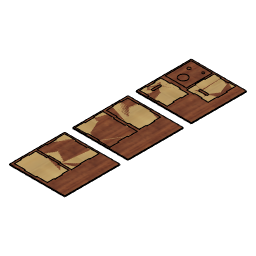
PLYO BOX v15 (Autodesk Fusion 360 design; units mm, degrees)
Autodesk Fusion 360 part; units mm, degrees
sketch "Sketch1" plane through (0, 0, 0) normal (0, 1, 0) x (1, 0, 0)
  line L0 (381, 304.8) -> (-381, 304.8)
  line L1 (-381, 304.8) -> (-381, -304.8)
  line L2 (-381, -304.8) -> (381, -304.8)
  line L3 (381, -304.8) -> (381, 304.8)
  line L4 (381, 304.8) -> (-381, -304.8) construction
  line L5 (-381, 304.8) -> (381, -304.8) construction
  line L6 (-127, 304.8) -> (127, 304.8)
  line L7 (127, 304.8) -> (127, 286.8)
  line L8 (127, 286.8) -> (-127, 286.8)
  line L9 (-127, 286.8) -> (-127, 304.8)
  line L10 (0, -304.8) -> (0, 304.8) construction
  line L11 (381, 0) -> (-381, 0) construction
  line L12 (127, -286.8) -> (-127, -286.8)
  line L13 (127, -304.8) -> (127, -286.8)
  line L14 (-127, -286.8) -> (-127, -304.8)
  line L15 (-381, -101.6) -> (-363, -101.6)
  line L16 (-363, -101.6) -> (-363, 101.6)
  line L17 (-363, 101.6) -> (-381, 101.6)
  line L18 (-381, 101.6) -> (-381, -101.6)
  line L19 (363, -101.6) -> (363, 101.6)
  line L20 (381, -101.6) -> (363, -101.6)
  line L21 (363, 101.6) -> (381, 101.6)
  dimension "Breedte" = 762
  dimension "Hoogte" = 609.6
  dimension "d3" = 254
  dimension "diktehout" = 18
  dimension "d5" = 203.2
  dimension "d6" = 18
  constraint horizontal L0
  constraint perpendicular L0 L1
  constraint parallel L0 L2
  constraint parallel L1 L3
  constraint coincident L4 origin
  constraint coincident L5 origin
  constraint horizontal L6
  constraint vertical L7
  constraint horizontal L8
  constraint vertical L9
  constraint coincident L0 L6.start
  constraint midpoint L2 L10.start
  constraint midpoint L0 L10.end
  constraint midpoint L3 L11.start
  constraint midpoint L1 L11.end
  constraint symmetric L7 L9 L10
  constraint symmetric L6.start L11 L14.end
  constraint symmetric L6.end L11 L13.start
  constraint symmetric L7.end L11 L12.start
  constraint symmetric L8.end L11 L12.end
  constraint horizontal L15
  constraint vertical L16
  constraint horizontal L17
  constraint vertical L18
  constraint coincident L1 L15.start
  constraint symmetric L11 L15 L17
  constraint symmetric L10 L15.start L20.start
  constraint symmetric L10 L15.end L19.start
  constraint symmetric L10 L16.end L19.end
  constraint symmetric L10 L17.end L21.end
  measures "Breedte" distance of L0.start L0.end
  measures "Hoogte" distance of L0.start L2.end
  measures "d3" distance of L7.end L8.end
  measures "diktehout" distance of L6.end L7.end
  measures "d5" distance of L15.end L16.end
  measures "d6" distance of L16.end L17.end
extrude "Extrude1" add sketch "Sketch1" along normal blind 18 contours L0 L1 L2 L3 L7 L8 L9 L12 L13 L14 L15 L16 L17 L19 L20 L21 makes body 1 in component "Voorkant"
sketch "Sketch1 (2)" plane through (381, 0, 0) normal (1, 0, 0) x (0, 1, 0) in component "zijkant"
  line L0 (0, 304.8) -> (0, 101.6)
  line L1 (0, 101.6) -> (18, 101.6)
  line L2 (18, 101.6) -> (18, 304.8)
  line L3 (18, 304.8) -> (0, 304.8)
  line L4 (18, 304.8) -> (-490, 304.8)
  line L5 (-490, 304.8) -> (-490, -304.8)
  line L6 (-490, -304.8) -> (18, -304.8)
  line L7 (18, -304.8) -> (18, 304.8)
  line L8 (18, 304.8) -> (0, 304.8)
  line L9 (0, 304.8) -> (0, -304.8)
  line L10 (0, -304.8) -> (18, -304.8)
  line L11 (18, -304.8) -> (18, 304.8)
  line L12 (18, -101.6) -> (0, -101.6)
  line L13 (18, 101.6) -> (0, 101.6)
  line L14 (-236, 304.8) -> (-236, -304.8) construction
  line L15 (-472, 304.8) -> (-472, -304.8)
  line L16 (-490, 101.6) -> (-472, 101.6)
  line L17 (-490, -101.6) -> (-472, -101.6)
  line L18 (-320.6667, 304.8) -> (-151.3333, 304.8)
  line L19 (-151.3333, 304.8) -> (-151.3333, 286.8)
  line L20 (-151.3333, 286.8) -> (-320.6667, 286.8)
  line L21 (-320.6667, 286.8) -> (-320.6667, 304.8)
  line L22 (18, 0) -> (-490, 0) construction
  line L23 (-151.3333, -286.8) -> (-320.6667, -286.8)
  line L24 (-320.6667, -286.8) -> (-320.6667, -304.8)
  line L25 (-151.3333, -304.8) -> (-151.3333, -286.8)
  dimension "d9" = 609.6
  dimension "Diepte" = 508
  dimension "d11" = 18
  dimension "d12" = 203.2
  dimension "d13" = 203.2
  dimension "d14" = 169.3333
  dimension "d15" = 18
  dimension "d92" = 0
  dimension "d93" = 0
  dimension "d94" = 0
  dimension "d95" = 0
  dimension "d104" = 0
  dimension "d105" = 0
  dimension "d106" = 0
  dimension "d107" = 0
  dimension "d156" = 0
  dimension "d157" = 0
  dimension "d158" = 0
  dimension "d159" = 0
  dimension "d172" = 0
  dimension "d173" = 0
  dimension "d174" = 0
  dimension "d175" = 0
  dimension "d180" = 0
  dimension "d181" = 0
  dimension "d182" = 0
  dimension "d183" = 0
  constraint horizontal L4
  constraint vertical L5
  constraint horizontal L6
  constraint vertical L7
  constraint coincident L2.end L3.start
  constraint horizontal L8
  constraint vertical L9
  constraint horizontal L10
  constraint vertical L11
  constraint coincident L6 L9.end
  constraint coincident L7 L12.start
  constraint coincident L9 L12.end
  constraint perpendicular L7 L12
  constraint coincident L1.end L2.start
  constraint coincident L0.end L1.start
  constraint midpoint L4 L14.start
  constraint midpoint L6 L14.end
  constraint symmetric L0.start L14 L15.start
  constraint symmetric L9.end L14 L15.end
  constraint symmetric L12.start L14 L17.start
  constraint symmetric L12.end L14 L17.end
  constraint symmetric L1.end L14 L16.start
  constraint symmetric L0.end L14 L16.end
  constraint horizontal L18
  constraint vertical L19
  constraint horizontal L20
  constraint vertical L21
  constraint coincident L4 L18.start
  constraint symmetric L14 L19 L21
  constraint midpoint L7 L22.start
  constraint midpoint L5 L22.end
  constraint symmetric L18.start L22 L24.end
  constraint symmetric L18.end L22 L25.start
  constraint symmetric L19.end L22 L23.start
  constraint symmetric L20.end L22 L23.end
  measures "d9" distance of L4.end L5.end
  measures "Diepte" distance of L2.end L4.end
  measures "d11" distance of L9.end L6.end
  measures "d12" distance of L4 L13
  measures "d13" distance of L10 L12
  measures "d14" distance of L19.end L20.end
  measures "d15" distance of L18.end L19.end
extrude "Extrude1'" add sketch "Sketch1 (2)" along normal blind 18 separate body contours L0 L4 L6 L9 L15 L19 L20 L21 L23 L24 L25 makes body 2 in component "Middenstuk"
extrude "Extrude1''" add sketch "Sketch1 (2)" against normal blind 18 separate body contours L0 L4 L6 L9 L15 L19 L20 L21 L23 L24 L25 | L1 L7 L9 L11 L12 L13 | L5 L15 L16 L17 makes body 3 in component "zijkant"
sketch "Sketch1 (3)" plane through (0, 0, -304.8) normal (0, 0, -1) x (1, 0, 0) in component "Onderkant"
  line L0 (-127, 0) -> (-381, 0)
  line L1 (-381, 0) -> (-381, -18)
  line L2 (-381, -18) -> (-127, -18)
  line L3 (-127, -18) -> (-127, 0)
  line L4 (381, -18) -> (-381, -18)
  line L5 (-381, -18) -> (-381, 490)
  line L6 (-381, 490) -> (381, 490)
  line L7 (381, 490) -> (381, -18)
  line L8 (363, 0) -> (-363, 0)
  line L9 (-363, 0) -> (-363, 472)
  line L10 (-363, 472) -> (363, 472)
  line L11 (363, 472) -> (363, 0)
  line L12 (127, 472) -> (127, 490)
  line L13 (-363, 151.3333) -> (-381, 151.3333)
  line L14 (-363, 320.6667) -> (-381, 320.6667)
  line L15 (-127, 472) -> (-127, 490)
  line L16 (0, -18) -> (0, 490) construction
  line L17 (-381, 236) -> (381, 236) construction
  line L18 (-127, 0) -> (-127, -18)
  line L19 (127, 0) -> (127, -18)
  line L20 (363, 151.3333) -> (381, 151.3333)
  line L21 (363, 320.6667) -> (381, 320.6667)
  point P0 (381, -18)
  dimension "d18" = 508
  dimension "d19" = 762
  dimension "d20" = 18
  dimension "d22" = 254
  dimension "d23" = 169.3333
  dimension "d60" = 0
  dimension "d61" = 0
  dimension "d62" = 0
  dimension "d63" = 0
  dimension "d72" = 0
  dimension "d73" = 0
  dimension "d74" = 0
  dimension "d75" = 0
  dimension "d80" = 0
  dimension "d81" = 0
  dimension "d82" = 0
  dimension "d83" = 0
  dimension "d132" = 0
  dimension "d133" = 0
  dimension "d134" = 0
  dimension "d135" = 0
  dimension "d140" = 0
  dimension "d141" = 0
  dimension "d142" = 0
  dimension "d143" = 0
  dimension "d148" = 0
  dimension "d149" = 0
  dimension "d150" = 0
  dimension "d151" = 0
  dimension "d164" = 0
  dimension "d165" = 0
  dimension "d166" = 0
  dimension "d167" = 0
  dimension "d188" = 0
  dimension "d189" = 0
  dimension "d190" = 0
  dimension "d191" = 0
  dimension "d196" = 0
  dimension "d197" = 0
  dimension "d198" = 0
  dimension "d199" = 0
  dimension "d220" = 0
  dimension "d221" = 0
  dimension "d222" = 0
  dimension "d223" = 0
  constraint horizontal L4
  constraint vertical L5
  constraint horizontal L6
  constraint vertical L7
  constraint coincident P0 L4.start
  constraint coincident L10 L12.start
  constraint coincident L6 L12.end
  constraint perpendicular L6 L12
  constraint coincident L9 L13.start
  constraint coincident L5 L13.end
  constraint perpendicular L5 L13
  constraint coincident L9 L14.start
  constraint coincident L5 L14.end
  constraint perpendicular L5 L14
  constraint coincident L10 L15.start
  constraint coincident L6 L15.end
  constraint perpendicular L6 L15
  constraint midpoint L4 L16.start
  constraint midpoint L6 L16.end
  constraint midpoint L5 L17.start
  constraint midpoint L7 L17.end
  constraint symmetric L13 L14 L17
  constraint symmetric L12 L15 L16
  constraint symmetric L12.start L17 L19.start
  constraint symmetric L12.end L17 L19.end
  constraint symmetric L15.start L17 L0.start
  constraint symmetric L15.end L17 L2.end
  constraint symmetric L13.start L16 L20.start
  constraint symmetric L13.end L16 L20.end
  constraint symmetric L14.start L16 L21.start
  constraint symmetric L14.end L16 L21.end
  measures "d18" distance of L1.end L5.end
  measures "d19" distance of L5.end L6.end
  measures "d22" distance of L12 L15
  measures "d23" distance of L13 L14
extrude "Extrude1'''" add sketch "Sketch1 (3)" against normal blind 18 separate body contours L3 L4 L8 L18 L19 | L0 L8 L9 L10 L11 | L5 L9 L13 L14 | L7 L11 L20 L21 | L6 L10 L12 L15 makes body 4 in component "Onderkant"
extrude "Extrude2" cut 2 faces at (387, -421.5556, -304.8) (387, -100.8889, -304.8) along direction (0, 0, -1) up to surface end surface through (381, -151.3333, -286.8) normal (0, 0, -1) offset 0 on bodies 2 bodies 2 in component "Middenstuk"
extrude "Extrude3" cut 2 faces at (387, -371.1111, 304.8) (387, -50.4444, 304.8) along direction (0, 0, 1) up to surface end surface through (381, -151.3333, 286.8) normal (0, 0, 1) offset 0 on bodies 2 bodies 2 in component "Middenstuk"
sketch "Sketch1 (4)" plane through (0, 0, 0) normal (0, 0, 1) x (1, 0, 0) in component "Houtplaat"
  line L0 (0, 0) -> (1220, 0)
  line L1 (1220, 0) -> (1220, -1220)
  line L2 (1220, -1220) -> (0, -1220)
  line L3 (0, -1220) -> (0, 0)
  dimension "d32" = 1220
  dimension "d33" = 1220
  dimension "d40" = 0
  dimension "d41" = 0
  dimension "d42" = 0
  dimension "d43" = 0
  dimension "d52" = 0
  dimension "d53" = 0
  dimension "d54" = 0
  dimension "d55" = 0
  dimension "d64" = 0
  dimension "d65" = 0
  dimension "d66" = 0
  dimension "d67" = 0
  dimension "d76" = 0
  dimension "d77" = 0
  dimension "d78" = 0
  dimension "d79" = 0
  dimension "d84" = 0
  dimension "d85" = 0
  dimension "d86" = 0
  dimension "d87" = 0
  dimension "d96" = 0
  dimension "d97" = 0
  dimension "d98" = 0
  dimension "d99" = 0
  dimension "d108" = 0
  dimension "d109" = 0
  dimension "d110" = 0
  dimension "d111" = 0
  dimension "d120" = 0
  dimension "d121" = 0
  dimension "d122" = 0
  dimension "d123" = 0
  dimension "d128" = 0
  dimension "d129" = 0
  dimension "d130" = 0
  dimension "d131" = 0
  dimension "d136" = 0
  dimension "d137" = 0
  dimension "d138" = 0
  dimension "d139" = 0
  dimension "d144" = 0
  dimension "d145" = 0
  dimension "d146" = 0
  dimension "d147" = 0
  dimension "d152" = 0
  dimension "d153" = 0
  dimension "d154" = 0
  dimension "d155" = 0
  dimension "d160" = 0
  dimension "d161" = 0
  dimension "d162" = 0
  dimension "d163" = 0
  dimension "d168" = 0
  dimension "d169" = 0
  dimension "d170" = 0
  dimension "d171" = 0
  dimension "d176" = 0
  dimension "d177" = 0
  dimension "d178" = 0
  dimension "d179" = 0
  dimension "d184" = 0
  dimension "d185" = 0
  dimension "d186" = 0
  dimension "d187" = 0
  dimension "d192" = 0
  dimension "d193" = 0
  dimension "d194" = 0
  dimension "d195" = 0
  dimension "d200" = 0
  dimension "d201" = 0
  dimension "d202" = 0
  dimension "d203" = 0
  dimension "d224" = 0
  dimension "d225" = 0
  dimension "d226" = 0
  dimension "d227" = 0
  constraint horizontal L0
  constraint vertical L1
  constraint horizontal L2
  constraint vertical L3
  constraint coincident L0.start L3.end
  measures "d32" distance of L0.start L2.end
  measures "d33" distance of L1.end L2.end
extrude "Extrude1''''" add sketch "Sketch1 (4)" along normal blind 18 separate body makes body 5 in component "Houtplaat"
sketch "Sketch2" plane through (381, 0, 0) normal (1, 0, 0) x (0, 1, 0)
  line L0 (18, -101.6) -> (18, 101.6)
  line L1 (18, 101.6) -> (0, 101.6)
  line L2 (0, 101.6) -> (0, 304.8)
  line L3 (0, 304.8) -> (-151.3333, 304.8)
  line L4 (-151.3333, 304.8) -> (-151.3333, 286.8)
  line L5 (-151.3333, 286.8) -> (-320.6667, 286.8)
  line L6 (-320.6667, 286.8) -> (-320.6667, 304.8)
  line L7 (-320.6667, 304.8) -> (-472, 304.8)
  line L8 (-472, 304.8) -> (-472, 101.6)
  line L9 (-472, 101.6) -> (-490, 101.6)
  line L10 (-490, 101.6) -> (-490, -101.6)
  line L11 (-490, -101.6) -> (-472, -101.6)
  line L12 (-472, -101.6) -> (-472, -304.8)
  line L13 (-472, -304.8) -> (-320.6667, -304.8)
  line L14 (-320.6667, -304.8) -> (-320.6667, -286.8)
  line L15 (-320.6667, -286.8) -> (-151.3333, -286.8)
  line L16 (-151.3333, -286.8) -> (-151.3333, -304.8)
  line L17 (-151.3333, -304.8) -> (0, -304.8)
  line L18 (0, -304.8) -> (0, -101.6)
  line L19 (0, -101.6) -> (18, -101.6)
  line L20 (-311, 141.8) -> (-161, 141.8)
  arc A0 (-161, 141.8) -> (-161, 191.8) centre (-161, 166.8) ccw
  line L21 (-161, 191.8) -> (-311, 191.8)
  arc A1 (-311, 191.8) -> (-311, 141.8) centre (-311, 166.8) ccw
  line L22 (-311, 166.8) -> (-161, 166.8) construction
  point P0 (-236, 166.8)
  dimension "d268" = 50
  dimension "d269" = 120
  constraint tangent L20 A0
  constraint tangent A0 L21
  constraint parallel L20 L21
  constraint tangent L21 A1
  constraint tangent L20 A1
  constraint parallel L5 L22
  constraint midpoint L22 P0
  measures "d268" diameter of A0
  measures "d269" distance of L5 P0
extrude "Extrude2'" cut sketch "Sketch2" against normal blind 50 contours L20 A0 L21 A1 bodies 3 in component "zijkant"
sketch "Sketch3" plane through (27, 0, 0) normal (1, 0, 0) x (0, 1, 0)
  line L0 (0, 286.8) -> (-472, 286.8)
  line L1 (-472, 286.8) -> (-472, -286.8)
  line L2 (-472, -286.8) -> (0, -286.8)
  line L3 (0, -286.8) -> (0, 286.8)
  circle A0 centre (-236, -121.8) radius 92.5
  circle A1 centre (-347, 116.8) radius 35
  circle A2 centre (-105, 186.8) radius 25
  line L4 (-236, -286.8) -> (-236, 286.8) construction
  dimension "d272" = 185
  dimension "d273" = 70
  dimension "d274" = 50
  dimension "d275" = 165
  dimension "d276" = 125
  dimension "d277" = 170
  dimension "d278" = 105
  dimension "d279" = 100
  constraint midpoint L2 L4.start
  constraint midpoint L0 L4.end
  constraint coincident A0.centre L4
  measures "d272" diameter of A0
  measures "d273" diameter of A1
  measures "d274" diameter of A2
  measures "d275" distance of L2 A0.centre
  measures "d276" distance of L1 A1.centre
  measures "d277" distance of L0 A1.centre
  measures "d278" distance of L3 A2.centre
  measures "d279" distance of L0 A2.centre
extrude "Extrude4" cut sketch "Sketch3" against normal up to surface (18 mm away) contours A0 | A1 | A2 sketch seen with x (1, 0, 0) y (0, 1, 0) z (0, 0, 1) at (372, 0, 0) bodies 2 in component "Middenstuk"
ref_plane "WorkPlane1" through (27, -236, 0) normal (1, 0, 0) x (0, 0, -1) in component "Laser Path - Middenstuk - Body1"
sketch "Path Offsets" plane through (27, 0, 0) normal (1, 0, 0) x (0, 0, -1) in component "Laser Path - Middenstuk - Body1"
  circle A0 centre (121.8, -236) radius 92.5
  circle A1 centre (-116.8, -347) radius 35
  circle A2 centre (-186.8, -105) radius 25
  line L0 (-286.8, 0) -> (-286.8, -472)
  line L1 (-286.8, -472) -> (286.8, -472)
  line L2 (286.8, -472) -> (286.8, 0)
  line L3 (286.8, 0) -> (-286.8, 0)
  line L4 (-286.8, -472) -> (286.8, -472)
  line L5 (286.8, -472) -> (286.8, 0)
  line L6 (286.8, 0) -> (-286.8, 0)
  line L7 (-286.8, 0) -> (-286.8, -472)
  dimension "d292" = 0
  measures "d292" distance of L1
sketch "Perimeter" plane through (27, -236, 0) normal (1, 0, 0) x (0, 0, -1) in component "Laser Path - Middenstuk - Body1"
  line L0 (286.8, 236) -> (-286.8, 236)
  line L1 (-286.8, 236) -> (-286.8, -236)
  line L2 (-286.8, -236) -> (286.8, -236)
  line L3 (286.8, -236) -> (286.8, 236)
sketch "Cutouts" plane through (27, -236, 0) normal (1, 0, 0) x (0, 0, -1) in component "Laser Path - Middenstuk - Body1"
  circle A0 centre (121.8, 0) radius 92.5
  circle A1 centre (-116.8, -111) radius 35
  circle A2 centre (-186.8, 131) radius 25
component "Voorkant" placed x (1, 0, 0) y (0, 0, 1) z (0, -1, 0) at (409, -1735.2, 0)
component "zijkant" placed x (0, 0, 1) y (0, 1, 0) z (-1, 0, 0) at (330, 702, -363)
component "Onderkant" placed x (1, 0, 0) y (0, 1, 0) z (0, 0, 1) at (409, -2083, 304.8)
component "Onderkant" placed x (1, 0, 0) y (0, 1, 0) z (0, 0, 1) at (406, -48, 304.8)
component "zijkant" placed x (0, 0, 1) y (-1, 0, 0) z (0, -1, 0) at (539, 1064.8, -363)
component "Middenstuk" placed x (0, 0, 1) y (1, 0, 0) z (0, 1, 0) at (498.4898, 1080.7872, -381.277)
component "Voorkant" placed x (1, 0, 0) y (0, 0, 1) z (0, -1, 0) at (406, -885.2, 0)
component "Houtplaat" placed x (1, 0, 0) y (0, 1, 0) z (0, 0, 1) at (0, 0, 0)
component "Laser Path - Middenstuk - Body1" placed x (1, 0, 0) y (0, 1, 0) z (0, 0, 1) at (0, 0, 0)
component "Houtplaat" placed x (1, 0, 0) y (0, 1, 0) z (0, 0, 1) at (0, -1400, 0)
component "Houtplaat" placed x (1, 0, 0) y (0, 1, 0) z (0, 0, 1) at (0, 1400, 0)
equation "d3 = Breedte / 3"
equation "d5 = Hoogte / 3"
equation "d6 = diktehout"
equation "d7 = diktehout"
equation "d9 = Hoogte"
equation "d11 = diktehout"
equation "d13 = Hoogte / 3"
equation "d14 = Diepte / 3"
equation "d15 = diktehout"
equation "d16 = -diktehout"
equation "d18 = Diepte"
equation "d19 = Breedte"
equation "d20 = diktehout"
equation "d22 = Breedte / 3"
equation "d23 = Diepte / 3"
equation "d24 = -diktehout"
equation "d26 = diktehout"
equation "d33 = 2440 mm / 2"
equation "offset = 0.00 mm"
